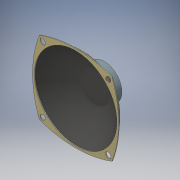
# Autodesk Inventor part: Nathan_Speaker
Saved by Autodesk Inventor 2016 (Build 200138000, 138)
## iProperties
Created: 2018-09-26
Part Number: Nathan_Speaker
Material: Generic
Document SubType Name: Modeling
Designer: Student
Density: 1 g/cm^3
Appearance: Default
Author: Student
Autodesk Inventor part; units mm, degrees
ref_plane "XZ Plane" through (0, 0, 0) normal (0, 1, 0) x (-1, 0, 0)
sketch "Sketch1" plane through (0, 0, 0) normal (0, 0, 1) x (1, 0, 0)
  circle A0 centre (-38.862, -38.862) radius 37.338
  arc A1 (-5.9943, -5.9943) -> (-71.7297, -5.9943) centre (-38.862, -93.1073) ccw
  arc A2 (-5.9943, -71.7297) -> (-5.9943, -5.9943) centre (-93.1073, -38.862) ccw
  arc A3 (-71.7297, -71.7297) -> (-5.9943, -71.7297) centre (-38.862, 15.3833) ccw
  arc A4 (-71.7297, -5.9943) -> (-71.7297, -71.7297) centre (15.3833, -38.862) ccw
  arc A5 (-7.3413, -7.3413) -> (-11.113, -11.113) centre (-8.8594, -9.595) ccw
  arc A6 (-11.113, -11.113) -> (-7.3413, -7.3413) centre (-9.595, -8.8594) ccw
  arc A7 (-66.611, -11.113) -> (-70.3827, -7.3413) centre (-68.8646, -9.595) ccw
  arc A8 (-70.3827, -7.3413) -> (-66.611, -11.113) centre (-68.129, -8.8594) ccw
  arc A9 (-11.113, -66.611) -> (-7.3413, -70.3827) centre (-8.8594, -68.129) ccw
  arc A10 (-7.3413, -70.3827) -> (-11.113, -66.611) centre (-9.595, -68.8646) ccw
  arc A11 (-70.3827, -70.3827) -> (-66.611, -66.611) centre (-68.8646, -68.129) ccw
  arc A12 (-66.611, -66.611) -> (-70.3827, -70.3827) centre (-68.129, -68.8646) ccw
  point P0 (0, 0)
  constraints: 24 point on circle, 13 centre point
extrude "Extrusion1" add sketch "Sketch1" along normal blind 0.635
ref_plane "Work Plane1" through (0, 0, -25.4) normal (0, 0, -1) x (-1, 0, 0)
sketch "Sketch2" plane through (0, 0, -25.4) normal (0, 0, -1) x (-1, 0, 0)
  circle A0 centre (38.862, -38.862) radius 37.338 projected
  circle A1 centre (38.862, -38.862) radius 15.875
  point P0 (0, 0)
  dimension "d19" = 31.75
  constraints: 1 centre point, 1 coincident
  measures "d19" diameter of A1
extrude "Extrusion2" add sketch "Sketch2" against normal blind 8.89 contours A1
ref_plane "Work Plane2" through (-38.862, 0, 0) normal (1, 0, 0) x (0, 1, 0)
sketch "Sketch6" plane through (-38.862, 0, 0) normal (1, 0, 0) x (0, 1, 0)
  line L0 (-22.987, -16.51) -> (-54.737, -16.51) projected
  arc A0 (-22.987, -16.51) -> (0, 0) centre (-35.8743, 25.6906) ccw
  arc A1 (-77.724, 0) -> (-54.737, -16.51) centre (-41.8497, 25.6906) ccw
  line L1 (-54.737, -16.51) -> (-52.197, -16.51)
  line L2 (-22.987, -16.51) -> (-25.527, -16.51)
  line L3 (-1.524, 0) -> (-76.2, 0) projected
  arc A2 (-76.2, 0) -> (-52.197, -16.51) centre (-39.2568, 28.0064) ccw
  line L4 (-77.724, 0) -> (-76.2, 0)
  line L5 (-71.7297, 0) -> (-77.724, 0) projected
  line L6 (-38.862, -16.51) -> (-38.862, 9.6565)
  dimension "d23" = 2.54
  dimension "d24" = 2.54
  constraints: 8 end point, 6 point on circle, 3 centre point, 2 point on line, 1 collinear, 1 midpoint, 1 vertical
  measures "d23" distance of L0.end L1.end
  measures "d24" distance of L0.start L2.end
revolve "Revolution1" add sketch "Sketch6" angle 360 about axis through (-38.862, -38.862, -16.51) along (0, 0, 1) contours L0 A1 L4 A2
body "Solid1"
